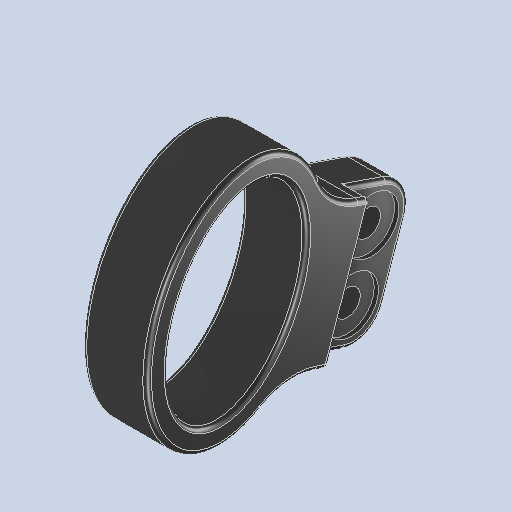
# Autodesk Inventor part: TorsoFrontBumper
Saved by Autodesk Inventor 2024.2 (Build 282272000, 272)
## iProperties
Created: 2024-01-21
Part Number: TorsoFrontBumper
Material: ABS Plastic
Document SubType Name: Modeling
Designer: Masato Kubotera
Density: 1.06 g/cm^3
Appearance: Glossy - Black
Mass: 18.7145 g
Surface Area: 72.9359 cm^2
Volume: 17.6552 cm^3
Catalog Web Link: https://www.poly-maker.jp/polyflex-tpu90.html
Author: Masato Kubotera
Autodesk Inventor part; units mm, degrees
ref_plane "YZ Plane" through (0, 0, 0) normal (1, 0, 0) x (0, 1, 0)
ref_plane "XZ Plane" through (0, 0, 0) normal (0, 1, 0) x (-1, 0, 0)
ref_plane "XY Plane" through (0, 0, 0) normal (0, 0, 1) x (1, 0, 0)
derived "TorsoSideFrame.ipt"
sketch "Sketch5" plane through (0, 0, 0) normal (0, 1, 0) x (-1, 0, 0)
  ellipse E0 centre (-84.0749, 16.6972) end of major axis (-76.7401, 37.9681) minor radius 15 projected
  ellipse E1 centre (-84.0749, 16.6972) end of major axis (-93.0397, -9.3006) minor radius 20 projected
  line L0 (-63.4041, 25.9649) -> (-37.3775, 16.9903) projected
  line L1 (-47.4832, -12.3163) -> (-73.5098, -3.3416) projected
  line L2 (-37.3775, 16.9903) -> (-47.4832, -12.3163) projected
  line L3 (-48.2759, 36) -> (-65, -12.5) projected
  point P0 (0, 0)
  point P1 (-52.5931, -1.8275)
  point P2 (-47.8663, 11.8804)
  point P3 (-63.0819, -6.9375)
  point P4 (-52.9762, 22.3691)
  constraints: 1 other
extrude "Extrusion2" add sketch "Sketch5" against normal blind 10
extrude "Extrusion5" add sketch "Sketch5" along normal blind 5 contours E1 | E1 L0 L3 L1
hole "Hole3" at (52.5931, 0, -1.8275) at (47.8663, 0, 11.8804) direction (0, -1, 0) diameter 6 end through all counterbore diameter 12.5 counterbore depth 1
fillet "Fillet9" radius 15 4 edges at (63.4041, -5, 25.9649) (63.4041, 2.5, 25.9649) (73.5098, -5, -3.3416) (73.5098, 2.5, -3.3416)
fillet "Fillet10" radius 1 17 edges at (91.4097, -10, -4.5737) (102.9824, -10, 23.217) (91.4097, 5, -4.5737) (42.4304, -10, 2.337) (56.713, -10, -9.1336) (46.6073, -10, 20.1729) (52.9762, 2.5, 22.3691) (63.0819, 2.5, -6.9375) (45.1768, 0, 19.6797) (55.2826, 0, -9.6269) (42.4304, 0, 2.337) (54.4066, 5, 22.8624) (102.9824, 5, 23.217) (72.3744, 5, -5.211) (64.5123, 5, -6.4442) (61.3578, 5, 26.7371) (58.029, 5, 7.7158)
fillet "Fillet11" radius 7.5 2 edges at (37.3775, -5, 16.9903) (47.4832, -5, -12.3163)
sketch "Sketch1" plane through (0, 0, 0) normal (0, 1, 0) x (-1, 0, 0)
  circle A0 centre (0, 0) radius 18.75 projected
  line L0 (0, 0) -> (0, -161.5) projected
  circle A1 centre (0, 0) radius 29 construction
  line L1 (0, 0) -> (0, 36) projected
  line L2 (0, 36) -> (-48.2759, 36) projected
  line L3 (-65, -12.5) -> (-65, -106.5) projected
  line L4 (-50, -161.5) -> (-35, -161.5) projected
  line L5 (-35, -161.5) -> (-35, -166.5) projected
  line L6 (-35, -166.5) -> (-10, -166.5) projected
  line L7 (-10, -166.5) -> (-10, -161.5) projected
  line L8 (-10, -161.5) -> (0, -161.5) projected
  line L9 (-60, -40.225) -> (-65, -40.225) projected
  line L10 (-44, -161.5) -> (-44, -155.5) construction
  line L11 (-22.5, -166.5) -> (-22.5, -161.5) construction
  arc A2 (-7, -161.5) -> (-10, -161.5) centre (-8.5, -161.5) ccw projected
  arc A3 (-35, -161.5) -> (-38, -161.5) centre (-36.5, -161.5) ccw projected
  line L12 (-65, -12.5) -> (-60, -12.5) construction
  line L13 (-60, -12.5) -> (-60, -101.5) construction
  line L14 (-62.5, -12.5) -> (-62.5, -101.5) construction
  line L15 (-65, -40.25) -> (-60, -40.25) construction
  arc A4 (-60, -43.225) -> (-60, -40.225) centre (-60, -41.725) ccw projected
  line L16 (-60, -106.5) -> (0, -106.5) construction
  line L17 (-60, -101.5) -> (0, -101.5) construction
  line L18 (-60, -104) -> (-18.75, -104) construction
  line L19 (-9.95, -106.55) -> (-27.55, -106.55) projected
  line L20 (-27.55, -106.55) -> (-27.55, -101.45) projected
  line L21 (-27.55, -101.45) -> (-9.95, -101.45) projected
  line L22 (-9.95, -101.45) -> (-9.95, -106.55) projected
  line L23 (-9.95, -106.55) -> (-27.55, -101.45) construction
  line L24 (-27.55, -106.55) -> (-9.95, -101.45) construction
  line L25 (-27.5, -101.5) -> (-27.5, -106.5) construction
  arc A5 (-24.55, -101.45) -> (-27.55, -101.45) centre (-26.05, -101.45) ccw projected
  arc A6 (-27.55, -106.55) -> (-24.55, -106.55) centre (-26.05, -106.55) ccw projected
  line L26 (-22.5, -71.5) -> (-42.5, -71.5) construction
  line L27 (-42.5, -71.5) -> (-42.5, -91.5) construction
  line L28 (-42.5, -91.5) -> (-22.5, -91.5) construction
  line L29 (-22.5, -91.5) -> (-22.5, -71.5) construction
  line L30 (-22.5, -71.5) -> (-42.5, -91.5) construction
  line L31 (-42.5, -71.5) -> (-22.5, -91.5) construction
  line L32 (-45, -69) -> (-20, -69) construction
  line L33 (-20, -69) -> (-20, -94) construction
  line L34 (-20, -94) -> (-45, -94) construction
  line L35 (-45, -94) -> (-45, -69) construction
  line L36 (-45, -69) -> (-20, -94) construction
  line L37 (-20, -69) -> (-45, -94) construction
  line L38 (-50, 31) -> (0, 31) construction
  line L39 (-38.05, 31.05) -> (-13.95, 31.05) projected
  line L40 (-13.95, 31.05) -> (-13.95, 25.95) projected
  line L41 (-13.95, 25.95) -> (-38.05, 25.95) projected
  line L42 (-38.05, 25.95) -> (-38.05, 31.05) projected
  line L43 (-38.05, 31.05) -> (-13.95, 25.95) construction
  line L44 (-13.95, 31.05) -> (-38.05, 25.95) construction
  line L45 (-38.05, 28.5) -> (-13.95, 28.5) construction
  line L46 (-38, 31) -> (-38, 26) construction
  line L47 (-26, 31.05) -> (-26, 25.95) construction
  line L48 (-14, 31) -> (-14, 26) construction
  arc A7 (-35.05, 31.05) -> (-38.05, 31.05) centre (-36.55, 31.05) ccw projected
  arc A8 (-38.05, 25.95) -> (-35.05, 25.95) centre (-36.55, 25.95) ccw projected
  arc A9 (-13.95, 31.05) -> (-16.95, 31.05) centre (-15.45, 31.05) ccw projected
  arc A10 (-16.95, 25.95) -> (-13.95, 25.95) centre (-15.45, 25.95) ccw projected
  line L49 (-46.0671, -156.5) -> (-3.5, -156.5) projected
  arc A11 (-47.9578, -155.152) -> (-46.0671, -156.5) centre (-46.0671, -154.5) ccw projected
  arc A12 (-3.5, -156.5) -> (-1.5, -154.5) centre (-3.5, -154.5) ccw projected
  line L50 (-56, -100.25) -> (-31.1254, -100.25) projected
  circle A13 centre (-41.25, -65.25) radius 2 construction
  line L51 (-1.5, -63.25) -> (-56, -63.25) projected
  line L52 (0, 0) -> (-29, 0) construction
  line L53 (-60, -107.75) -> (-31.1254, -107.75) projected
  arc A14 (-29.4336, -108.6833) -> (-23.3669, -109.5167) centre (-26.05, -106.55) ccw projected
  line L54 (-1.5, -154.5) -> (-1.5, -109.75) projected
  arc A15 (-1.5, -109.75) -> (-3.5, -107.75) centre (-3.5, -109.75) ccw projected
  arc A16 (-29.4336, -108.6833) -> (-31.1254, -107.75) centre (-31.1254, -109.75) ccw projected
  circle A17 centre (-33.5, -104) radius 1.75 construction
  arc A18 (-22.0254, -109) -> (-23.3669, -109.5167) centre (-22.0254, -111) ccw projected
  line L55 (-18.75, -101.45) -> (-18.75, -106.55) construction
  arc A19 (-31.1254, -100.25) -> (-29.4336, -99.3167) centre (-31.1254, -98.25) ccw projected
  arc A20 (-23.3669, -98.4833) -> (-29.4336, -99.3167) centre (-26.05, -101.45) ccw projected
  arc A21 (-23.3669, -98.4833) -> (-22.0254, -99) centre (-22.0254, -97) ccw projected
  line L56 (-10, -101.5) -> (-10, -106.5) construction
  arc A22 (-12.95, -106.55) -> (-9.95, -106.55) centre (-11.45, -106.55) ccw projected
  arc A23 (-6.3746, -107.75) -> (-8.0664, -108.6833) centre (-6.3746, -109.75) ccw projected
  arc A24 (-14.1331, -109.5167) -> (-15.4746, -109) centre (-15.4746, -111) ccw projected
  arc A25 (-14.1331, -109.5167) -> (-8.0664, -108.6833) centre (-11.45, -106.55) ccw projected
  arc A26 (-9.95, -101.45) -> (-12.95, -101.45) centre (-11.45, -101.45) ccw projected
  arc A27 (-15.4746, -99) -> (-14.1331, -98.4833) centre (-15.4746, -97) ccw projected
  arc A28 (-8.0664, -99.3167) -> (-14.1331, -98.4833) centre (-11.45, -101.45) ccw projected
  arc A29 (-8.0664, -99.3167) -> (-6.3746, -100.25) centre (-6.3746, -98.25) ccw projected
  line L57 (-22.0254, -99) -> (-15.4746, -99) projected
  line L58 (-22.0254, -109) -> (-15.4746, -109) projected
  line L59 (-6.3746, -107.75) -> (-3.5, -107.75) projected
  line L60 (-6.3746, -100.25) -> (-3.5, -100.25) projected
  arc A30 (-3.5, -100.25) -> (-1.5, -98.25) centre (-3.5, -98.25) ccw projected
  line L61 (-41.25, -65.25) -> (-36.25, -65.25) construction
  line L62 (-60, -43.225) -> (-60, -87.275) projected
  line L63 (-60, -65.25) -> (-65, -65.25) construction
  line L64 (-65, -90.25) -> (-60, -90.25) construction
  arc A31 (-60, -90.275) -> (-60, -87.275) centre (-60, -88.775) ccw projected
  line L65 (-60, -90.275) -> (-65, -90.275) projected
  line L66 (-60, -101.5) -> (-65, -101.5) construction
  line L67 (-1.5, -22.4499) -> (-1.5, -63.25) projected
  line L68 (-56, -67.25) -> (-1.5, -67.25) projected
  line L69 (-1.5, -67.25) -> (-1.5, -98.25) projected
  line L70 (-56, -63.25) -> (-56, -45.4999) projected
  circle A32 centre (-32.5, -81.5) radius 10 projected
  line L71 (-56, -67.25) -> (-56, -100.25) projected
  circle A33 centre (-32.5, -81.5) radius 11 projected
  arc A34 (-14.0872, 17.5443) -> (-22.2374, 3.4277) centre (0, 0) ccw projected
  arc A35 (-22.2374, -3.4277) -> (-14.0872, -17.5443) centre (0, 0) ccw projected
  arc A36 (-8.1502, -20.972) -> (-1.5, -22.4499) centre (0, 0) ccw projected
  arc A37 (-22.2374, 3.4277) -> (-22.2374, -3.4277) centre (-24.75, 0) ccw projected
  line L72 (-48.2759, 36) -> (-65, -12.5) projected
  arc A38 (-42.9869, 36) -> (-50, 31) centre (-42.9869, 28.5817) ccw projected
  line L73 (-75.1102, 42.6949) -> (-93.0397, -9.3006) construction
  ellipse E0 centre (-84.0749, 16.6972) end of major axis (-76.7401, 37.9681) minor radius 15 construction
  ellipse E1 centre (-84.0749, 16.6972) end of major axis (-93.0397, -9.3006) minor radius 20 construction
  line L74 (-75.1102, 42.6949) -> (-76.7401, 37.9681) construction
  line L75 (-105, 43.5) -> (-105, 11.4504) construction
  line L76 (-84.0749, 16.6972) -> (-58.029, 7.7158) construction
  line L77 (-63.4041, 25.9649) -> (-37.3775, 16.9903) construction
  line L78 (-37.3775, 16.9903) -> (-47.4832, -12.3163) construction
  line L79 (-47.4832, -12.3163) -> (-73.5098, -3.3416) construction
  line L80 (-79.9787, 43.5) -> (-105, 43.5) construction
  line L81 (-45.1768, 19.6797) -> (-55.2826, -9.6269) construction
  circle A39 centre (-47.8663, 11.8804) radius 6.25 construction
  circle A40 centre (-52.5931, -1.8275) radius 6.25 construction
  line L82 (-1, 13.5) -> (-28, 13.5) construction
  line L83 (-28, 13.5) -> (-28, -13.5) construction
  line L84 (-28, -13.5) -> (-1, -13.5) construction
  line L85 (-1, -13.5) -> (-1, 13.5) construction
  line L86 (-1, 13.5) -> (-28, -13.5) construction
  line L87 (-28, 13.5) -> (-1, -13.5) construction
  line L88 (0, -65.25) -> (-65, -65.25) construction
  line L89 (-50, -161.5) -> (-65, -118) projected
  line L90 (-16.326, 23) -> (-48.5275, 23) projected
  arc A41 (-16.326, 23) -> (-14.0872, 17.5443) centre (-12.375, 21.4341) ccw projected
  line L91 (-65, -106.5) -> (-65, -118) projected
  arc A42 (-56, -45.4999) -> (-60, -36.225) centre (-60, -41.725) ccw projected
  arc A43 (-46.8371, 5.7157) -> (-50.3902, 17.5981) centre (-47.8663, 11.8804) ccw projected
  arc A44 (-46.8371, 5.7157) -> (-47.983, 2.3925) centre (-46.5078, 3.743) ccw projected
  arc A45 (-58.1048, -4.7743) -> (-47.983, 2.3925) centre (-52.5931, -1.8275) ccw projected
  line L92 (-48.5275, 23) -> (-50.3902, 17.5981) projected
  line L93 (-38, 26) -> (-14, 26) construction
  line L94 (-58.1048, -4.7743) -> (-60, -10.2703) projected
  line L95 (-60, -36.225) -> (-60, -10.2703) projected
  line L96 (-39.0921, -23.3529) -> (-39.0921, -46.6256) construction
  line L97 (-54.0921, -23.3529) -> (-54.0921, -46.6256) construction
  line L98 (-39.0921, -23.3529) -> (-54.0921, -23.3529) construction
  line L99 (-39.0921, -46.6256) -> (-54.0921, -46.6256) construction
  line L100 (-16.326, -23) -> (-48.5275, -23) projected
  arc A46 (-14.0872, -17.5443) -> (-16.326, -23) centre (-12.375, -21.4341) ccw projected
  line L101 (-47.9578, -155.152) -> (-50.3902, -148.0981) projected
  arc A47 (-50.3902, -148.0981) -> (-46.8371, -136.2157) centre (-47.8663, -142.3804) ccw projected
  arc A48 (-47.983, -132.8925) -> (-46.8371, -136.2157) centre (-46.5078, -134.243) ccw projected
  arc A49 (-47.983, -132.8925) -> (-58.1048, -125.7257) centre (-52.5931, -128.6725) ccw projected
  line L102 (-58.1048, -125.7257) -> (-60, -120.2297) projected
  line L103 (-60, -120.2297) -> (-60, -107.75) projected
  point P0 (-16.05, -9.6933)
  point P1 (-12.375, -21.4341)
  point P2 (12.375, -21.4341)
  point P3 (24.75, 0)
  point P4 (12.375, 21.4341)
  point P5 (-26, 28.5)
  point P6 (0, -130.75)
  point P7 (0, -158.0887)
  point P8 (-44, 28.5)
  point P9 (-61.4811, -94)
  point P10 (-1.5, -156.5)
  point P11 (-5, -161.5)
  point P12 (-29.8658, -107.75)
  point P13 (-30.0089, -107.1221)
  point P14 (-7.6342, -107.75)
  point P15 (-38, 28.5)
  point P16 (-14.5, 0)
  point P17 (-1, 0)
  point P18 (0, 22.5)
  point P19 (-62.5, -30.25)
  point P20 (-62.5, -100.25)
  constraints: 5 other
body "Solid2"
